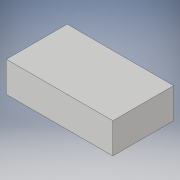
# Autodesk Inventor part: Part35
Saved by Autodesk Inventor 2019.4 (Build 234330000, 330)
## iProperties
Created: 2020-02-19
Part Number: Part35
Material: Generic
Document SubType Name: Modeling
Designer: Niran
Density: 1 g/cm^3
Appearance: Default
Author: Niran
Autodesk Inventor part; units mm, degrees
ref_plane "YZ Plane" through (0, 0, 0) normal (1, 0, 0) x (0, 1, 0)
ref_plane "XZ Plane" through (0, 0, 0) normal (0, 1, 0) x (-1, 0, 0)
ref_plane "XY Plane" through (0, 0, 0) normal (0, 0, 1) x (1, 0, 0)
sketch "Sketch1" plane through (0, 0, 0) normal (0, 1, 0) x (-1, 0, 0)
  line L0 (0, 0) -> (-35, 0)
  line L1 (-35, 0) -> (-35, -20)
  line L2 (-35, -20) -> (0, -20)
  line L3 (0, -20) -> (0, 0)
  dimension "d0" = 35
  dimension "d1" = 20
  constraints: 8 end point, 2 parallel, 1 horizontal, 1 perpendicular
  measures "d0" distance of L2.end L1.end
  measures "d1" distance of L1.end L0.end
extrude "Extrusion1" add sketch "Sketch1" along normal blind 10
body "Solid1"
